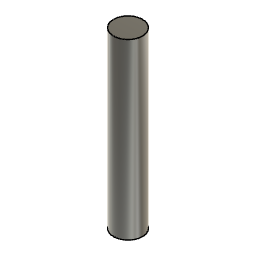
中轴(须打印2份) v1 (Autodesk Fusion 360 design; units mm, degrees)
Autodesk Fusion 360 part; units mm, degrees
sketch "草图1" plane through (0, 0, 0) normal (0, 0, 1) x (1, 0, 0)
  circle A0 centre (3.7639, 9.9475) radius 0.5
  dimension "d1" = 1
  measures "d1" diameter of A0
extrude "拉伸1" add sketch "草图1" along normal blind 6
